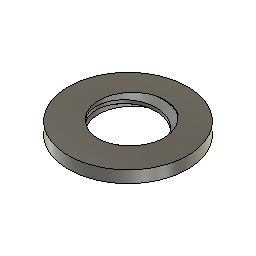
rotoforgeender3gantryassembly v4 v4 (Autodesk Fusion 360 archive; units mm, degrees)
design "pneumaticfittingspacer"
Autodesk Fusion 360 part; units mm, degrees
sketch "Sketch1" plane through (0, 0, 0) normal (0, 0, 1) x (1, 0, 0)
  circle A0 centre (0, 0) radius 5
  circle A1 centre (0, 0) radius 2.5
  dimension "d1" = 10
  dimension "d2" = 5
  constraint coincident A0.centre A1.centre
  measures "d1" diameter of A0
  measures "d2" diameter of A1
extrude "Extrude1" add sketch "Sketch1" along normal blind 1
thread "Thread1" "ISO Metric profile 6.0 M6x1 6H" major diameter 6.147 minor diameter 5.035 pitch 1 angle 60 modelled right hand crest width 0.2748 on face at (2.4969, -0.1246, 0.6667) crest through (2.5175, 0, 0.25)
